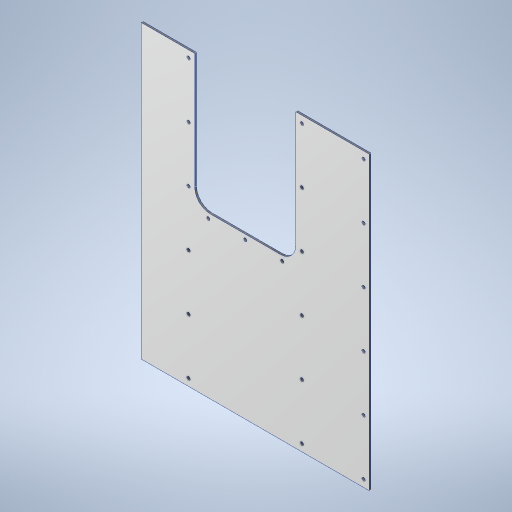
# Autodesk Inventor part: Side Internal Side Panel R2
Saved by Autodesk Inventor 2024 (Build 280153000, 153)
## iProperties
Created: 2024-09-28
Part Number: Side Internal Side Panel R2
Material: Generic
Document SubType Name: Modeling
Designer: Ishaan
Density: 1 g/cm^3
Appearance: Default
Author: Ishaan
Autodesk Inventor part; units mm, degrees
note: some values were not read from the file. Chosen so that the rebuilt part matches the saved one: hole positions of "Sketch Driven Pattern1".
ref_plane "YZ Plane" through (0, 0, 0) normal (1, 0, 0) x (0, 1, 0)
ref_plane "XZ Plane" through (0, 0, 0) normal (0, 1, 0) x (-1, 0, 0)
ref_plane "XY Plane" through (0, 0, 0) normal (0, 0, 1) x (1, 0, 0)
sketch "Sketch1" plane through (0, 0, 0) normal (0, 0, 1) x (1, 0, 0)
  line L0 (185, -236.5) -> (-185, -236.5)
  line L1 (-185, -236.5) -> (-185, 236.5)
  line L2 (-185, 236.5) -> (185, 236.5)
  line L3 (185, 236.5) -> (185, -236.5)
  line L4 (185, -236.5) -> (-185, 236.5) construction
  line L5 (-185, -236.5) -> (185, 236.5) construction
  point P0 (0, 0)
  dimension "d0" = 370
  dimension "d1" = 473
  constraints: 12 end point, 2 midpoint, 2 parallel, 1 horizontal, 1 perpendicular
  measures "d0" distance of L1.end L2.end
  measures "d1" distance of L0.end L1.end
extrude "Extrusion1" add sketch "Sketch1" along normal mid plane 3
extrude "Extrusion2" cut sketch "Sketch1" along normal mid plane 2.9
extrude "Extrusion3" add sketch "Sketch1" along normal mid plane 2.9 separate body
sketch "Sketch6" plane through (0, 0, 1.5) normal (0, 0, 1) x (1, 0, 0)
  line L0 (176, -225) -> (-176, -225) construction
  line L1 (-176, -225) -> (-176, 225) construction
  line L2 (-176, 225) -> (176, 225) construction
  line L3 (176, 225) -> (176, -225) construction
  line L4 (176, -225) -> (-176, 225) construction
  line L5 (-176, -225) -> (176, 225) construction
  point P0 (-176, 135)
  point P1 (-176, 45)
  point P2 (-176, -45)
  point P3 (-176, -135)
  point P4 (0, 0)
  point P5 (0, 0)
  point P6 (176, 135)
  point P7 (176, 45)
  point P8 (176, -45)
  point P9 (176, -135)
  point P10 (176, -225)
  dimension "d49" = 352
  dimension "d52" = 90
  dimension "d71" = 450
  dimension "d77" = 90
  constraints: 12 end point, 4 coincident, 2 parallel, 2 vertical, 1 horizontal, 1 midpoint, 1 perpendicular, 10 other
  measures "d49" distance of L1.end L2.end
  measures "d52" distance of point (-176, 225) point (-176, 135)
  measures "d71" distance between parallel lines of L0 L2
  measures "d77" distance of point (176, 225) point (176, 135)
hole "Hole4" at (176, 225, 1.5) at (176, 135, 1.5) at (176, 45, 1.5) at (176, -45, 1.5) at (176, -135, 1.5) at (176, -225, 1.5) direction (0, 0, -1) diameter 5.3 end through all bodies 1 2
sketch "Sketch8" plane through (0, 0, 1.5) normal (0, 0, 1) x (1, 0, 0)
  circle A0 centre (176, 225) radius 2.75 projected
  point P0 (-108, 225)
  point P1 (76, 225)
  dimension "d73" = 100
  dimension "d74" = 184
  constraints: 2 horizontal alignment, 1 coincident
  measures "d73" distance of point (176, 225) point (76, 225)
  measures "d74" distance of point (76, 225) point (-108, 225)
pattern_sketch "Sketch Driven Pattern1" of "Hole4" from (176, 225, 1.5) bodies 1 2 copies at (-108, 225, 1.5) at (76, 225, 1.5)
sketch "Sketch9" plane through (0, 0, 1.5) normal (0, 0, 1) x (1, 0, 0)
  line L0 (-98, 237.5) -> (66, 237.5)
  line L1 (66, 237.5) -> (66, 48.5)
  line L2 (41, 23.5) -> (-73, 23.5)
  line L3 (-98, 48.5) -> (-98, 237.5)
  circle A0 centre (-108, 225) radius 2.65 projected
  circle A1 centre (76, 225) radius 2.65 projected
  line L4 (185, 236.5) -> (-185, 236.5) projected
  line L5 (-76, 15.5) -> (44, 15.5) construction
  arc A2 (-98, 48.5) -> (-73, 23.5) centre (-73, 48.5) ccw
  arc A3 (41, 23.5) -> (66, 48.5) centre (41, 48.5) ccw
  point P0 (0, 0)
  point P1 (66, 23.5)
  point P2 (-16, 23.5)
  point P3 (-16, 15.5)
  point P4 (-16, 15.5)
  point P5 (66, 236.5)
  point P6 (-98, 236.5)
  dimension "d82" = 10
  dimension "d83" = 10
  dimension "d84" = 1
  dimension "d85" = 214
  dimension "d86" = 120
  dimension "d87" = 8
  dimension "d98" = 25
  constraints: 10 end point, 4 point on circle, 4 tangent, 3 coincident, 2 centre point, 2 horizontal, 2 midpoint, 2 parallel, 2 point on line, 1 equal radius, 1 perpendicular, 1 vertical alignment
  measures "d82" distance from line of L3 A0.centre
  measures "d83" distance from line of A1.centre L1
  measures "d84" distance between parallel lines of L0 L4
  measures "d85" distance of L0.end point (66, 23.5)
  measures "d86" distance of L5.start L5.end
  measures "d87" distance between parallel lines of L2 L5
  measures "d98" radius of A2
hole "Hole5" at (-76, 15.5, 1.5) at (-16, 15.5, 1.5) at (44, 15.5, 1.5) direction (0, 0, -1) diameter 5.3 end through all bodies 1 2
extrude "Extrusion6" cut sketch "Sketch9" against normal through all contours L4 L1 A3 L2 A2 L3 bodies 1 2
equation "\"d77\" = d52"
equation "\"d83\" = d82"
